Autodesk Fusion 360 part; units mm, degrees
(part 2 of 2)
  line L958 (271, 254, 0.0025) -> (271, 239, 0.0025)
  line L959 (271, 239, 0.0025) -> (256, 239, 0.0025)
  line L960 (1, 271, 0.0025) -> (16, 271, 0.0025)
  line L961 (1, 256, 0.0025) -> (1, 271, 0.0025)
  line L962 (16, 271, 0.0025) -> (16, 256, 0.0025)
  line L963 (16, 256, 0.0025) -> (1, 256, 0.0025)
  line L964 (18, 271, 0.0025) -> (33, 271, 0.0025)
  line L965 (18, 256, 0.0025) -> (18, 271, 0.0025)
  line L966 (33, 271, 0.0025) -> (33, 256, 0.0025)
  line L967 (33, 256, 0.0025) -> (18, 256, 0.0025)
  line L968 (35, 271, 0.0025) -> (50, 271, 0.0025)
  line L969 (35, 256, 0.0025) -> (35, 271, 0.0025)
  line L970 (50, 271, 0.0025) -> (50, 256, 0.0025)
  line L971 (50, 256, 0.0025) -> (35, 256, 0.0025)
  line L972 (52, 271, 0.0025) -> (67, 271, 0.0025)
  line L973 (52, 256, 0.0025) -> (52, 271, 0.0025)
  line L974 (67, 271, 0.0025) -> (67, 256, 0.0025)
  line L975 (67, 256, 0.0025) -> (52, 256, 0.0025)
  line L976 (69, 271, 0.0025) -> (84, 271, 0.0025)
  line L977 (69, 256, 0.0025) -> (69, 271, 0.0025)
  line L978 (84, 271, 0.0025) -> (84, 256, 0.0025)
  line L979 (84, 256, 0.0025) -> (69, 256, 0.0025)
  line L980 (86, 271, 0.0025) -> (101, 271, 0.0025)
  line L981 (86, 256, 0.0025) -> (86, 271, 0.0025)
  line L982 (101, 271, 0.0025) -> (101, 256, 0.0025)
  line L983 (101, 256, 0.0025) -> (86, 256, 0.0025)
  line L984 (103, 271, 0.0025) -> (118, 271, 0.0025)
  line L985 (103, 256, 0.0025) -> (103, 271, 0.0025)
  line L986 (118, 271, 0.0025) -> (118, 256, 0.0025)
  line L987 (118, 256, 0.0025) -> (103, 256, 0.0025)
  line L988 (120, 271, 0.0025) -> (135, 271, 0.0025)
  line L989 (120, 256, 0.0025) -> (120, 271, 0.0025)
  line L990 (135, 271, 0.0025) -> (135, 256, 0.0025)
  line L991 (135, 256, 0.0025) -> (120, 256, 0.0025)
  line L992 (137, 271, 0.0025) -> (152, 271, 0.0025)
  line L993 (137, 256, 0.0025) -> (137, 271, 0.0025)
  line L994 (152, 271, 0.0025) -> (152, 256, 0.0025)
  line L995 (152, 256, 0.0025) -> (137, 256, 0.0025)
  line L996 (154, 271, 0.0025) -> (169, 271, 0.0025)
  line L997 (154, 256, 0.0025) -> (154, 271, 0.0025)
  line L998 (169, 271, 0.0025) -> (169, 256, 0.0025)
  line L999 (169, 256, 0.0025) -> (154, 256, 0.0025)
  line L1000 (171, 271, 0.0025) -> (186, 271, 0.0025)
  line L1001 (171, 256, 0.0025) -> (171, 271, 0.0025)
  line L1002 (186, 271, 0.0025) -> (186, 256, 0.0025)
  line L1003 (186, 256, 0.0025) -> (171, 256, 0.0025)
  line L1004 (188, 271, 0.0025) -> (203, 271, 0.0025)
  line L1005 (188, 256, 0.0025) -> (188, 271, 0.0025)
  line L1006 (203, 271, 0.0025) -> (203, 256, 0.0025)
  line L1007 (203, 256, 0.0025) -> (188, 256, 0.0025)
  line L1008 (205, 271, 0.0025) -> (220, 271, 0.0025)
  line L1009 (205, 256, 0.0025) -> (205, 271, 0.0025)
  line L1010 (220, 271, 0.0025) -> (220, 256, 0.0025)
  line L1011 (220, 256, 0.0025) -> (205, 256, 0.0025)
  line L1012 (222, 271, 0.0025) -> (237, 271, 0.0025)
  line L1013 (222, 256, 0.0025) -> (222, 271, 0.0025)
  line L1014 (237, 271, 0.0025) -> (237, 256, 0.0025)
  line L1015 (237, 256, 0.0025) -> (222, 256, 0.0025)
  line L1016 (239, 271, 0.0025) -> (254, 271, 0.0025)
  line L1017 (239, 256, 0.0025) -> (239, 271, 0.0025)
  line L1018 (254, 271, 0.0025) -> (254, 256, 0.0025)
  line L1019 (254, 256, 0.0025) -> (239, 256, 0.0025)
  line L1020 (256, 271, 0.0025) -> (271, 271, 0.0025)
  line L1021 (256, 256, 0.0025) -> (256, 271, 0.0025)
  line L1022 (271, 271, 0.0025) -> (271, 256, 0.0025)
  line L1023 (271, 256, 0.0025) -> (256, 256, 0.0025)
  dimension "d44" = 15
  dimension "d45" = 15
  dimension "d46" = 1
  dimension "d47" = 1
move_body "Verschieben2" bodies 1 to x (1, 0, 0) y (0, 1, 0) z (0, 0, 1) at (0, 0, -1)
sketch "Skizze8" plane through (0, 0, 0) normal (0, 0, 1) x (1, 0, 0)
  line L0 (2.5, 271) -> (14.5, 271)
  line L1 (14.5, 271) -> (14.5, 1)
  line L2 (14.5, 1) -> (2.5, 1)
  line L3 (2.5, 1) -> (2.5, 271)
  line L4 (31.5, 271) -> (31.5, 1)
  line L5 (19.5, 1) -> (19.5, 271)
  line L6 (19.5, 271) -> (31.5, 271)
  line L7 (31.5, 1) -> (19.5, 1)
  line L8 (48.5, 271) -> (48.5, 1)
  line L9 (36.5, 1) -> (36.5, 271)
  line L10 (36.5, 271) -> (48.5, 271)
  line L11 (48.5, 1) -> (36.5, 1)
  line L12 (65.5, 271) -> (65.5, 1)
  line L13 (53.5, 1) -> (53.5, 271)
  line L14 (53.5, 271) -> (65.5, 271)
  line L15 (65.5, 1) -> (53.5, 1)
  line L16 (82.5, 271) -> (82.5, 1)
  line L17 (70.5, 1) -> (70.5, 271)
  line L18 (70.5, 271) -> (82.5, 271)
  line L19 (82.5, 1) -> (70.5, 1)
  line L20 (99.5, 271) -> (99.5, 1)
  line L21 (87.5, 1) -> (87.5, 271)
  line L22 (87.5, 271) -> (99.5, 271)
  line L23 (99.5, 1) -> (87.5, 1)
  line L24 (116.5, 271) -> (116.5, 1)
  line L25 (104.5, 1) -> (104.5, 271)
  line L26 (104.5, 271) -> (116.5, 271)
  line L27 (116.5, 1) -> (104.5, 1)
  line L28 (133.5, 271) -> (133.5, 1)
  line L29 (121.5, 1) -> (121.5, 271)
  line L30 (121.5, 271) -> (133.5, 271)
  line L31 (133.5, 1) -> (121.5, 1)
  line L32 (150.5, 271) -> (150.5, 1)
  line L33 (138.5, 1) -> (138.5, 271)
  line L34 (138.5, 271) -> (150.5, 271)
  line L35 (150.5, 1) -> (138.5, 1)
  line L36 (167.5, 271) -> (167.5, 1)
  line L37 (155.5, 1) -> (155.5, 271)
  line L38 (155.5, 271) -> (167.5, 271)
  line L39 (167.5, 1) -> (155.5, 1)
  line L40 (184.5, 271) -> (184.5, 1)
  line L41 (172.5, 1) -> (172.5, 271)
  line L42 (172.5, 271) -> (184.5, 271)
  line L43 (184.5, 1) -> (172.5, 1)
  line L44 (201.5, 271) -> (201.5, 1)
  line L45 (189.5, 1) -> (189.5, 271)
  line L46 (189.5, 271) -> (201.5, 271)
  line L47 (201.5, 1) -> (189.5, 1)
  line L48 (218.5, 271) -> (218.5, 1)
  line L49 (206.5, 1) -> (206.5, 271)
  line L50 (206.5, 271) -> (218.5, 271)
  line L51 (218.5, 1) -> (206.5, 1)
  line L52 (235.5, 271) -> (235.5, 1)
  line L53 (223.5, 1) -> (223.5, 271)
  line L54 (223.5, 271) -> (235.5, 271)
  line L55 (235.5, 1) -> (223.5, 1)
  line L56 (252.5, 271) -> (252.5, 1)
  line L57 (240.5, 1) -> (240.5, 271)
  line L58 (240.5, 271) -> (252.5, 271)
  line L59 (252.5, 1) -> (240.5, 1)
  line L60 (269.5, 271) -> (269.5, 1)
  line L61 (257.5, 1) -> (257.5, 271)
  line L62 (257.5, 271) -> (269.5, 271)
  line L63 (269.5, 1) -> (257.5, 1)
  dimension "d57" = 270
  dimension "d58" = 12
  dimension "d59" = 2.5
  dimension "d60" = 1
  dimension "d63" = 255
  dimension "d64" = 0
  constraint horizontal L0
  constraint vertical L1
  constraint horizontal L2
  constraint vertical L3
  measures "d57" distance of L0.end L1.end
  measures "d58" distance of L0.start L0.end
  measures "d59" distance of origin L3
  measures "d60" distance of origin L2
sketch "Skizze9" plane through (0, 0, 0) normal (0, 0, 1) x (1, 0, 0)
  line L0 (1, 11) -> (271, 11)
  line L1 (271, 11) -> (271, 6)
  line L2 (271, 6) -> (1, 6)
  line L3 (1, 6) -> (1, 11)
  line L4 (1, 266) -> (271, 266)
  line L5 (271, 261) -> (1, 261)
  line L6 (271, 266) -> (271, 261)
  line L7 (1, 261) -> (1, 266)
  dimension "d67" = 270
  dimension "d68" = 5
  dimension "d69" = 1
  dimension "d70" = 6
  dimension "d71" = 270
  dimension "d72" = 5
  constraint horizontal L0
  constraint vertical L1
  constraint horizontal L2
  constraint vertical L3
  constraint horizontal L4
  constraint vertical L6
  constraint horizontal L5
  constraint vertical L7
  measures "d67" distance of L1.end L2.end
  measures "d68" distance of L0.start L2.end
  measures "d69" distance of origin L3
  measures "d70" distance of origin L2
  measures "d71" distance of L5.start L5.end
  measures "d72" distance of L5.end L4.start
extrude "Extrusion8" cut sketch "Skizze7" along normal blind 10 contours L0 L1 L2 L3 | L4 L5 L6 L7 | L8 L9 L10 L11 | L12 L13 L14 L15 | L16 L17 L18 L19 | L20 L21 L22 L23 | L24 L25 L26 L27 | L28 L29 L30 L31 | L32 L33 L34 L35 | L36 L37 L38 L39 | L40 L41 L42 L43 | L44 L45 L46 L47 | L48 L49 L50 L51 | L52 L53 L54 L55 | L56 L57 L58 L59 | L60 L61 L62 L63 | L64 L65 L66 L67 | L68 L69 L70 L71 | L72 L73 L74 L75 | L76 L77 L78 L79 | L80 L81 L82 L83 | L84 L85 L86 L87 | L88 L89 L90 L91 | L92 L93 L94 L95 | L96 L97 L98 L99 | L100 L101 L102 L103 | L104 L105 L106 L107 | L108 L109 L110 L111 | L112 L113 L114 L115 | L116 L117 L118 L119 | L120 L121 L122 L123 | L124 L125 L126 L127 | L128 L129 L130 L131 | L132 L133 L134 L135 | L136 L137 L138 L139 | L140 L141 L142 L143 | L144 L145 L146 L147 | L148 L149 L150 L151 | L152 L153 L154 L155 | L156 L157 L158 L159 | L160 L161 L162 L163 | L164 L165 L166 L167 | L168 L169 L170 L171 | L172 L173 L174 L175 | L176 L177 L178 L179 | L180 L181 L182 L183 | L184 L185 L186 L187 | L188 L189 L190 L191 | L192 L193 L194 L195 | L196 L197 L198 L199 | L200 L201 L202 L203 | L204 L205 L206 L207 | L208 L209 L210 L211 | L212 L213 L214 L215 | L216 L217 L218 L219 | L220 L221 L222 L223 | L224 L225 L226 L227 | L228 L229 L230 L231 | L232 L233 L234 L235 | L236 L237 L238 L239 | L240 L241 L242 L243 | L244 L245 L246 L247 | L248 L249 L250 L251 | L252 L253 L254 L255 | L256 L257 L258 L259 | L260 L261 L262 L263 | L264 L265 L266 L267 | L268 L269 L270 L271 | L272 L273 L274 L275 | L276 L277 L278 L279 | L280 L281 L282 L283 | L284 L285 L286 L287 | L288 L289 L290 L291 | L292 L293 L294 L295 | L296 L297 L298 L299 | L300 L301 L302 L303 | L304 L305 L306 L307 | L308 L309 L310 L311 | L312 L313 L314 L315 | L316 L317 L318 L319 | L320 L321 L322 L323 | L324 L325 L326 L327 | L328 L329 L330 L331 | L332 L333 L334 L335 | L336 L337 L338 L339 | L340 L341 L342 L343 | L344 L345 L346 L347 | L348 L349 L350 L351 | L352 L353 L354 L355 | L356 L357 L358 L359 | L360 L361 L362 L363 | L364 L365 L366 L367 | L368 L369 L370 L371 | L372 L373 L374 L375 | L376 L377 L378 L379 | L380 L381 L382 L383 | L384 L385 L386 L387 | L388 L389 L390 L391 | L392 L393 L394 L395 | L396 L397 L398 L399 | L400 L401 L402 L403 | L404 L405 L406 L407 | L408 L409 L410 L411 | L412 L413 L414 L415 | L416 L417 L418 L419 | L420 L421 L422 L423 | L424 L425 L426 L427 | L428 L429 L430 L431 | L432 L433 L434 L435 | L436 L437 L438 L439 | L440 L441 L442 L443 | L444 L445 L446 L447 | L448 L449 L450 L451 | L452 L453 L454 L455 | L456 L457 L458 L459 | L460 L461 L462 L463 | L464 L465 L466 L467 | L468 L469 L470 L471 | L472 L473 L474 L475 | L476 L477 L478 L479 | L480 L481 L482 L483 | L484 L485 L486 L487 | L488 L489 L490 L491 | L492 L493 L494 L495 | L496 L497 L498 L499 | L500 L501 L502 L503 | L504 L505 L506 L507 | L508 L509 L510 L511 | L512 L513 L514 L515 | L516 L517 L518 L519 | L520 L521 L522 L523 | L524 L525 L526 L527 | L528 L529 L530 L531 | L532 L533 L534 L535 | L536 L537 L538 L539 | L540 L541 L542 L543 | L544 L545 L546 L547 | L548 L549 L550 L551 | L552 L553 L554 L555 | L556 L557 L558 L559 | L560 L561 L562 L563 | L564 L565 L566 L567 | L568 L569 L570 L571 | L572 L573 L574 L575 | L576 L577 L578 L579 | L580 L581 L582 L583 | L584 L585 L586 L587 | L588 L589 L590 L591 | L592 L593 L594 L595 | L596 L597 L598 L599 | L600 L601 L602 L603 | L604 L605 L606 L607 | L608 L609 L610 L611 | L612 L613 L614 L615 | L616 L617 L618 L619 | L620 L621 L622 L623 | L624 L625 L626 L627 | L628 L629 L630 L631 | L632 L633 L634 L635 | L636 L637 L638 L639 | L640 L641 L642 L643 | L644 L645 L646 L647 | L648 L649 L650 L651 | L652 L653 L654 L655 | L656 L657 L658 L659 | L660 L661 L662 L663 | L664 L665 L666 L667 | L668 L669 L670 L671 | L672 L673 L674 L675 | L676 L677 L678 L679 | L680 L681 L682 L683 | L684 L685 L686 L687 | L688 L689 L690 L691 | L692 L693 L694 L695 | L696 L697 L698 L699 | L700 L701 L702 L703 | L704 L705 L706 L707 | L708 L709 L710 L711 | L712 L713 L714 L715 | L716 L717 L718 L719 | L720 L721 L722 L723 | L724 L725 L726 L727 | L728 L729 L730 L731 | L732 L733 L734 L735 | L736 L737 L738 L739 | L740 L741 L742 L743 | L744 L745 L746 L747 | L748 L749 L750 L751 | L752 L753 L754 L755 | L756 L757 L758 L759 | L760 L761 L762 L763 | L764 L765 L766 L767 | L768 L769 L770 L771 | L772 L773 L774 L775 | L776 L777 L778 L779 | L780 L781 L782 L783 | L784 L785 L786 L787 | L788 L789 L790 L791 | L792 L793 L794 L795 | L796 L797 L798 L799 | L800 L801 L802 L803 | L804 L805 L806 L807 | L808 L809 L810 L811 | L812 L813 L814 L815 | L816 L817 L818 L819 | L820 L821 L822 L823 | L824 L825 L826 L827 | L828 L829 L830 L831 | L832 L833 L834 L835 | L836 L837 L838 L839 | L840 L841 L842 L843 | L844 L845 L846 L847 | L848 L849 L850 L851 | L852 L853 L854 L855 | L856 L857 L858 L859 | L860 L861 L862 L863 | L864 L865 L866 L867 | L868 L869 L870 L871 | L872 L873 L874 L875 | L876 L877 L878 L879 | L880 L881 L882 L883 | L884 L885 L886 L887 | L888 L889 L890 L891 | L892 L893 L894 L895 | L896 L897 L898 L899 | L900 L901 L902 L903 | L904 L905 L906 L907 | L908 L909 L910 L911 | L912 L913 L914 L915 | L916 L917 L918 L919 | L920 L921 L922 L923 | L924 L925 L926 L927 | L928 L929 L930 L931 | L932 L933 L934 L935 | L936 L937 L938 L939 | L940 L941 L942 L943 | L944 L945 L946 L947 | L948 L949 L950 L951 | L952 L953 L954 L955 | L956 L957 L958 L959 | L960 L961 L962 L963 | L964 L965 L966 L967 | L968 L969 L970 L971 | L972 L973 L974 L975 | L976 L977 L978 L979 | L980 L981 L982 L983 | L984 L985 L986 L987 | L988 L989 L990 L991 | L992 L993 L994 L995 | L996 L997 L998 L999 | L1000 L1001 L1002 L1003 | L1004 L1005 L1006 L1007 | L1008 L1009 L1010 L1011 | L1012 L1013 L1014 L1015 | L1016 L1017 L1018 L1019 | L1020 L1021 L1022 L1023 in plane through (0, 0, 0.0025) normal (0, 0, 1)
extrude "Extrusion9" cut sketch "Skizze8" along normal blind 2.5
extrude "Extrusion10" cut sketch "Skizze9" along normal blind 4
sketch "Skizze11" plane through (0, 0, 0) normal (0, 0, 1) x (1, 0, 0)
  line L0 (5, 4) -> (12, 4)
  line L1 (12, 4) -> (12, 2)
  line L2 (12, 2) -> (5, 2)
  line L3 (5, 2) -> (5, 4)
  line L4 (22, 4) -> (29, 4)
  line L5 (29, 4) -> (29, 2)
  line L6 (29, 2) -> (22, 2)
  line L7 (22, 2) -> (22, 4)
  line L8 (39, 4) -> (46, 4)
  line L9 (46, 4) -> (46, 2)
  line L10 (46, 2) -> (39, 2)
  line L11 (39, 2) -> (39, 4)
  line L12 (56, 4) -> (63, 4)
  line L13 (63, 4) -> (63, 2)
  line L14 (63, 2) -> (56, 2)
  line L15 (56, 2) -> (56, 4)
  line L16 (73, 4) -> (80, 4)
  line L17 (80, 4) -> (80, 2)
  line L18 (80, 2) -> (73, 2)
  line L19 (73, 2) -> (73, 4)
  line L20 (90, 4) -> (97, 4)
  line L21 (97, 4) -> (97, 2)
  line L22 (97, 2) -> (90, 2)
  line L23 (90, 2) -> (90, 4)
  line L24 (107, 4) -> (114, 4)
  line L25 (114, 4) -> (114, 2)
  line L26 (114, 2) -> (107, 2)
  line L27 (107, 2) -> (107, 4)
  line L28 (124, 4) -> (131, 4)
  line L29 (131, 4) -> (131, 2)
  line L30 (131, 2) -> (124, 2)
  line L31 (124, 2) -> (124, 4)
  line L32 (141, 4) -> (148, 4)
  line L33 (148, 4) -> (148, 2)
  line L34 (148, 2) -> (141, 2)
  line L35 (141, 2) -> (141, 4)
  line L36 (158, 4) -> (165, 4)
  line L37 (165, 4) -> (165, 2)
  line L38 (165, 2) -> (158, 2)
  line L39 (158, 2) -> (158, 4)
  line L40 (175, 4) -> (182, 4)
  line L41 (182, 4) -> (182, 2)
  line L42 (182, 2) -> (175, 2)
  line L43 (175, 2) -> (175, 4)
  line L44 (192, 4) -> (199, 4)
  line L45 (199, 4) -> (199, 2)
  line L46 (199, 2) -> (192, 2)
  line L47 (192, 2) -> (192, 4)
  line L48 (209, 4) -> (216, 4)
  line L49 (216, 4) -> (216, 2)
  line L50 (216, 2) -> (209, 2)
  line L51 (209, 2) -> (209, 4)
  line L52 (226, 4) -> (233, 4)
  line L53 (233, 4) -> (233, 2)
  line L54 (233, 2) -> (226, 2)
  line L55 (226, 2) -> (226, 4)
  line L56 (243, 4) -> (250, 4)
  line L57 (250, 4) -> (250, 2)
  line L58 (250, 2) -> (243, 2)
  line L59 (243, 2) -> (243, 4)
  line L60 (260, 4) -> (267, 4)
  line L61 (267, 4) -> (267, 2)
  line L62 (267, 2) -> (260, 2)
  line L63 (260, 2) -> (260, 4)
  dimension "d81" = 7
  dimension "d82" = 2
  dimension "d83" = 5
  dimension "d84" = 2
  dimension "d87" = 255
  dimension "d88" = 0
  constraint horizontal L0
  constraint vertical L1
  constraint horizontal L2
  constraint vertical L3
  measures "d81" distance of L0.start L0.end
  measures "d82" distance of L0.start L2.end
  measures "d83" distance of origin L3
  measures "d84" distance of origin L2
extrude "Extrusion11" cut sketch "Skizze11" against normal blind 3
